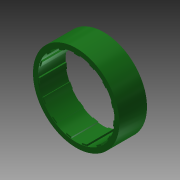
# Autodesk Inventor part: Automoblox TireTL
Saved by Autodesk Inventor 2015 (Build 190159000, 159)
## iProperties
Created: 2015-02-03
Part Number: Automoblox TireTL
Material: Generic
Document SubType Name: Modeling
Designer: PLTW-Stu-02
Density: 1 g/cm^3
Appearance: Smooth - Dark Forest Green
Author: PLTW-Stu-02
Autodesk Inventor part; units mm, degrees
ref_plane "YZ Plane" through (0, 0, 0) normal (1, 0, 0) x (0, 1, 0)
ref_plane "XZ Plane" through (0, 0, 0) normal (0, 1, 0) x (-1, 0, 0)
ref_plane "XY Plane" through (0, 0, 0) normal (0, 0, 1) x (1, 0, 0)
sketch "Sketch1" plane through (0, 0, 0) normal (0, 0, 1) x (1, 0, 0)
  arc A0 (34.6858, 43.8208) -> (31.9926, 43.8208) centre (33.3392, 24.5638) ccw
  circle A1 centre (33.3392, 24.5638) radius 20.066
  circle A2 centre (33.3392, 24.5638) radius 22.606
  line L0 (34.6858, 43.8208) -> (34.739, 44.581)
  line L1 (31.9926, 43.8208) -> (31.9395, 44.581)
  point P0 (0, 0)
  dimension "d0" = 38.608
  dimension "d3" = 0.762
  dimension "d4" = 2.54
  constraints: 4 end point, 4 point on circle, 3 centre point, 2 coincident
  measures "d0" diameter of A0
  measures "d3" radial gap between concentric circles of A1 A0
  measures "d4" radial gap between concentric circles of A1 A2
extrude "Extrusion2" add sketch "Sketch1" along normal mid plane 14.478
extrude "Extrusion3" add sketch "Sketch1" along normal mid plane 13.97 contours A0 L1 A1 L0 picked at (34.4103, 44.3421)
pattern_circular "Circular Pattern1" count 15 over 360 about axis through (33.3392, 24.5638, 0) along (0, 0, 1) of "Extrusion3"
body "Solid2"
